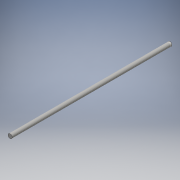
# Autodesk Inventor part: shaft
Saved by Autodesk Inventor 2016 (Build 200138000, 138)
## iProperties
Created: 2017-06-20
Part Number: shaft
Material: Generic
Document SubType Name: Modeling
Designer: M228544
Density: 1 g/cm^3
Appearance: Default
Author: M228544
Autodesk Inventor part; units mm, degrees
ref_plane "YZ Plane" through (0, 0, 0) normal (1, 0, 0) x (0, 1, 0)
ref_plane "XZ Plane" through (0, 0, 0) normal (0, 1, 0) x (-1, 0, 0)
ref_plane "XY Plane" through (0, 0, 0) normal (0, 0, 1) x (1, 0, 0)
sketch "Sketch1" plane through (0, 0, 0) normal (0, 1, 0) x (-1, 0, 0)
  circle A0 centre (0, 0) radius 7
  dimension "d0" = 14
  constraints: 1 centre point, 1 coincident
  measures "d0" diameter of A0
extrude "Extrusion1" add sketch "Sketch1" along normal blind 530
thread "Thread1" size "1/2-13 UNC" class "2A" standard "ANSI Unified Screw Threads" length 530 offset 5
body "Solid1"
